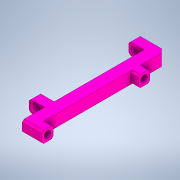
# Autodesk Inventor part: camadapter2
Saved by Autodesk Inventor 2020 (Build 240168000, 168)
## iProperties
Created: 2020-11-07
Part Number: camadapter2
Material: Generic
Document SubType Name: Modeling
Designer: alnwlsn
Density: 1 g/cm^3
Appearance: Default
Author: alnwlsn
Autodesk Inventor part; units mm, degrees
ref_plane "YZ Plane" through (0, 0, 0) normal (1, 0, 0) x (0, 1, 0)
ref_plane "XZ Plane" through (0, 0, 0) normal (0, 1, 0) x (-1, 0, 0)
ref_plane "XY Plane" through (0, 0, 0) normal (0, 0, 1) x (1, 0, 0)
sketch "Sketch1" plane through (0, 0, 0) normal (0, 1, 0) x (-1, 0, 0)
  line L0 (0, 0) -> (0, -6)
  line L1 (0, -6) -> (4, -6)
  line L2 (4, -6) -> (4, -50)
  line L3 (4, -50) -> (0, -50)
  line L4 (0, -50) -> (0, -56)
  line L5 (0, 0) -> (10, 0)
  line L6 (0, 0) -> (10, 0)
  line L7 (10, 0) -> (10, -11.5)
  line L8 (10, -11.5) -> (18, -11.5)
  line L9 (18, -11.5) -> (18, -16.5)
  line L10 (18, -16.5) -> (10, -16.5)
  line L11 (10, -16.5) -> (10, -63)
  line L12 (10, -63) -> (18, -63)
  line L13 (18, -63) -> (18, -68)
  line L14 (18, -68) -> (10, -68)
  line L15 (0, -56) -> (4, -56)
  line L16 (4, -56) -> (4, -68)
  line L17 (4, -68) -> (10, -68)
  point P0 (0, -3)
  point P1 (0, -53)
  dimension "d2" = 50
  dimension "d3" = 6
  dimension "d4" = 4
  dimension "d19" = 6
  dimension "d20" = 11.5
  dimension "d21" = 5
  dimension "d22" = 8
  dimension "d23" = 46.5
  constraints: 36 end point, 11 perpendicular, 7 point on line, 3 collinear, 3 horizontal, 2 midpoint, 1 vertical
  measures "d2" distance of point (0, -53) point (0, -3)
  measures "d3" distance between parallel lines of L5 L1
  measures "d4" distance between parallel lines of L0 L2
  measures "d19" distance between parallel lines of L7 L2
  measures "d20" distance of L6.end L7.end
  measures "d21" distance between parallel lines of L8 L10
  measures "d22" distance between parallel lines of L7 L9
  measures "d23" distance between parallel lines of L12 L10
extrude "Extrusion1" add sketch "Sketch1" along normal blind 6
sketch "Sketch4" plane through (0, 0, -50) normal (1, 0, 0) x (0, 0, -1)
  line L0 (-44, 0) -> (0, 0) projected
  line L1 (-50, 0) -> (-50, 6) projected
  line L2 (-44, 0) -> (-50, 6) construction
  circle A0 centre (-47, 3) radius 1.75
  line L3 (0, 0) -> (6, 0) projected
  line L4 (-44, 6) -> (0, 6) projected
  line L5 (6, 0) -> (0, 6) construction
  circle A1 centre (3, 3) radius 1.75
  dimension "d24" = 3.5
  constraints: 4 end point, 2 centre point, 2 midpoint, 1 equal radius
  measures "d24" diameter of A0
extrude "Extrusion4" cut sketch "Sketch4" against normal through all
chamfer "Chamfer2" distance 1 angle 45 8 edges at (-5, 6, 0) (-2, 6, -6) (-2, 0, -6) (-5, 0, 0) (-2, 0, -50) (-2, 6, -50) (-2, 0, -56) (-2, 6, -56)
chamfer "Chamfer3" distance 2 angle 45 1 edges at (-4, 3, -68)
sketch "Sketch5" plane through (-18, 0, -11.5) normal (0, 0, 1) x (1, 0, 0)
  circle A0 centre (3, 3) radius 3 construction
  line L0 (0, 6) -> (8, 6) projected
  line L1 (0, 0) -> (0, 6) projected
  line L2 (0, 0) -> (8, 0) projected
  circle A1 centre (3, 3) radius 1.75
  point P0 (18, 0)
  dimension "d33" = 3.5
  constraints: 3 tangent, 2 centre point, 1 coincident
  measures "d33" diameter of A1
chamfer "Chamfer4" distance 1 angle 45 4 edges at (-18, 0, -65.5) (-18, 6, -65.5) (-18, 0, -14) (-18, 6, -14)
extrude "Extrusion5" cut sketch "Sketch5" against normal through all
chamfer "Chamfer5" distance 1 angle 45 2 edges at (-16.75, 3, -11.5) (-16.75, 3, -68)
body "Solid1"
